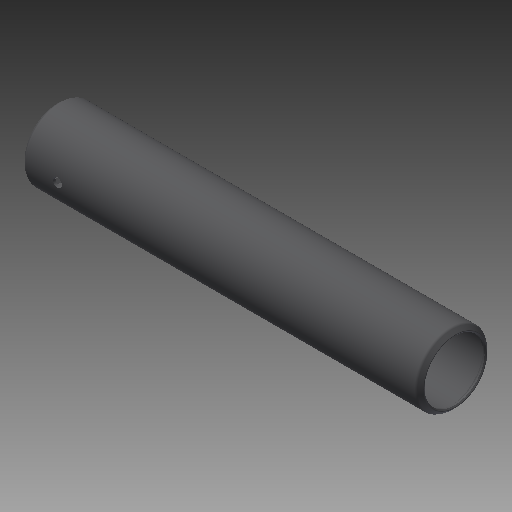
# Autodesk Inventor part: 01-2.6622
Saved by Autodesk Inventor 2017 (Build 210142000, 142)
## iProperties
Category: PARTsolutions
Company: BIMBA
Created: 2017-01-31
Part Number: 01-2.6622
Catalog Web Link: www.cadenas.de
Description: Tube-Original Line - Standard Air Cylinders
Vendor: BIMBA
Document SubType Name: Modeling
Designer: psAdmin
Manufacturer: BIMBA
Mass: 1.21411 g
Surface Area: 51.2105 cm^2
Volume: 1.21411 cm^3
Density: 1 g/cm^3
Material: Generic
Appearance: PSOLRGB-180-180-180
PSOL_IDENT_0: {$CADENAS_DATA\23d-libs\bimba\bimba\bimba_imperial\bimba_full_line\original_line_cylinders\standard_
PSOL_IDENT_1: air_cylinders\tube.prj},186 {VTYP=3D},{NB=01-2.6622},{LINA=01-2.6622},{NN=Tube},{DATE=09.11.2016 07:
PSOL_IDENT_2: 55:11},{GEOMDATE=18.02.2011 00:00:00},{VERSION=},{LINEID=20},{LINESUBID=-1},{WBVAR=MNT,ACTING,NR,L,F
PSOL_IDENT_3: OURHOLES,SR}  {NB=01-2.6622},{LINA=01-2.6622},{KT=DUMMY},{PN=01-2.6622},{BORE=0.43750000},{BOREPN=01
PSOL_IDENT_4: },{MNT=},{MNTALG='' , 'Front Nose' , 'BF' , 'Front Block' , 'BFT' , 'Front Trunnion'},{ACTING=},{ACT
PSOL_IDENT_5: INGALG= '' , 'Single Acting' , 'R' , 'Reverse/Double Acting' },{NR=},{NRALG= '' , 'Without Non-rotat
PSOL_IDENT_6: ing Rod' , 'NR' , 'With Non-rotating Rod' },{L=2.6620},{OD=0.4840},{ODN=0.4840},{ODP=0.7380},{ODB=0.
PSOL_IDENT_7: 0000},{ID=0.4465},{DV=0.00000000},{LV=0.00000000},{LV1=0.00000000},{G=0.0200},{FOURHOLES=2},{AA=0.25
PSOL_IDENT_8: 00},{BB=0.0620},{SR=},{SRALG= 'C' , 'Carbon Steel Rod' , 'SR' , '303 Stainless Steel Rod' , '' , '30
PSOL_IDENT_9: 3 Stainless Steel Rod'}
NN: Tube
NT: Original Line - Standard Air Cylinders
NB: 01-2.6622
NBSYN: $PN.
LINA: 01-2.6622
BORE: 7/16
BOREPN: 01
MNT: Front Nose
MNTALG: '' , 'Front Nose' , 'BF' , 'Front Block' , 'BFT' , 'Front Trunnion'
ACTING: Single Acting
NR: Without Non-rotating Rod
L: 2.6620
ODN: 0.4840
ODP: 0.7380
ODB: 0.0000
ID: 0.4465
DV: 0.00000000
LV: 0.00000000
LV1: 0.00000000
G: 0.0200
FOURHOLES: 2
AA: 0.2500
BB: 0.0620
SR: 303 Stainless Steel Rod
SUPPLIER: BIMBA
ARTICLENO: 01-2.6622
BOMINFO: 01-2.6622
CREATOR: CADENAS GmbH
Title: 01-2.6622
Author: Cadenas PARTsolutions
Comments: Original Line - Standard Air Cylinders
Autodesk Inventor part; units mm, degrees
sketch "Sketch_1" plane through (0, 0, 0) normal (0, 0, 1) x (1, 0, 0)
  line L0 (67.6148, 0) -> (0, 0)
  arc A0 (-0.3964, 5.4846) -> (-0.3964, 5.305) centre (-0.3066, 5.3948) ccw
  line L1 (-0.3964, 5.305) -> (-0.254, 5.1626)
  line L2 (-0.254, 5.1626) -> (0, 5.1626)
  line L3 (0, 5.1626) -> (0.508, 5.6706)
  line L4 (0.508, 5.6706) -> (67.1068, 5.6706)
  line L5 (67.1068, 5.6706) -> (67.6148, 5.1626)
  line L6 (67.6148, 5.1626) -> (67.8688, 5.1626)
  line L7 (67.8688, 5.1626) -> (68.0112, 5.305)
  arc A1 (68.0112, 5.305) -> (68.0112, 5.4846) centre (67.9214, 5.3948) ccw
  line L8 (68.0112, 5.4846) -> (67.4978, 5.998)
  arc A2 (67.4978, 5.998) -> (67.1385, 6.1468) centre (67.1385, 5.6388) ccw
  line L9 (67.1385, 6.1468) -> (0.4763, 6.1468)
  arc A3 (0.4763, 6.1468) -> (0.117, 5.998) centre (0.4763, 5.6388) ccw
  line L10 (0.117, 5.998) -> (-0.3964, 5.4846)
  constraints: 22 end point, 8 point on circle, 4 centre point
revolve "Revolution1" add sketch "Sketch_1" angle 360 about axis through (67.6148, 0, 0) along (1, 0, 0)
sketch "Sketch_4" plane through (0, 0, 0) normal (0, 0, 1) x (1, 0, 0)
  circle A0 centre (5.842, 0) radius 0.7874
  constraints: 1 centre point
extrude "Extrusion1" cut sketch "Sketch_4" along normal blind 6.1468
ref_plane "cp1_XY" through (33.8074, 6.1468, 0) normal (1, 0, 0) x (0, 0, -1)
ref_plane "cp1_YZ" through (33.8074, 6.1468, 0) normal (0, 0, -1) x (0, 1, 0)
ref_plane "cp1_ZX" through (33.8074, 6.1468, 0) normal (0, 1, 0) x (1, 0, 0)
ref_plane "cp2_XY" through (33.8074, 0, -6.1468) normal (1, 0, 0) x (0, 0, -1)
ref_plane "cp2_YZ" through (33.8074, 0, -6.1468) normal (0, 0, -1) x (0, 1, 0)
ref_plane "cp2_ZX" through (33.8074, 0, -6.1468) normal (0, 1, 0) x (1, 0, 0)
ref_plane "cp3_XY" through (33.8074, -6.1468, 0) normal (1, 0, 0) x (0, 0, -1)
ref_plane "cp3_YZ" through (33.8074, -6.1468, 0) normal (0, 0, -1) x (0, 1, 0)
ref_plane "cp3_ZX" through (33.8074, -6.1468, 0) normal (0, 1, 0) x (1, 0, 0)
ref_plane "cp4_XY" through (33.8074, 0, 6.1468) normal (1, 0, 0) x (0, 0, -1)
ref_plane "cp4_YZ" through (33.8074, 0, 6.1468) normal (0, 0, -1) x (0, 1, 0)
ref_plane "cp4_ZX" through (33.8074, 0, 6.1468) normal (0, 1, 0) x (1, 0, 0)
ref_plane "tube_front_XY" through (0, 0, 0) normal (1, 0, 0) x (0, 0, -1)
ref_plane "tube_front_YZ" through (0, 0, 0) normal (0, 0, -1) x (0, 1, 0)
ref_plane "tube_front_ZX" through (0, 0, 0) normal (0, 1, 0) x (1, 0, 0)
ref_plane "tube_rear_XY" through (67.6148, 0, 0) normal (1, 0, 0) x (0, 0, -1)
ref_plane "tube_rear_YZ" through (67.6148, 0, 0) normal (0, 0, -1) x (0, 1, 0)
ref_plane "tube_rear_ZX" through (67.6148, 0, 0) normal (0, 1, 0) x (1, 0, 0)
body "Solid1"
